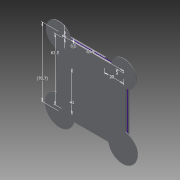
# Autodesk Inventor part: OuterCover
Saved by Autodesk Inventor 2014 SP1 (Build 180222100, 222)
## iProperties
Created: 2014-08-07
Part Number: OuterCover
Material: Generic
Document SubType Name: Modeling
Designer: Erin
Density: 1 g/cm^3
Appearance: Default
Author: Erin
Autodesk Inventor part; units mm, degrees
ref_plane "YZ Plane" through (0, 0, 0) normal (1, 0, 0) x (0, 1, 0)
ref_plane "XZ Plane" through (0, 0, 0) normal (0, 1, 0) x (-1, 0, 0)
ref_plane "XY Plane" through (0, 0, 0) normal (0, 0, 1) x (1, 0, 0)
sketch "Sketch1" plane through (0, 0, 0) normal (0, 1, 0) x (-1, 0, 0)
  line L0 (-31.75, 31.75) -> (31.75, 31.75)
  line L1 (31.75, 31.75) -> (31.75, -31.75)
  line L2 (31.75, -31.75) -> (-31.75, -31.75)
  line L3 (-31.75, -31.75) -> (-31.75, 31.75)
  line L4 (-31.75, 9.25) -> (31.75, 9.25) construction
  line L5 (-31.75, 26.75) -> (-11.75, 26.75) construction
  line L6 (-11.75, 26.75) -> (-11.75, 31.75) construction
  line L7 (32.35, 32.35) -> (-32.35, 32.35)
  line L8 (-32.35, 32.35) -> (-32.35, -32.35)
  line L9 (-32.35, -32.35) -> (32.35, -32.35)
  line L10 (32.35, -32.35) -> (32.35, 32.35)
  line L11 (-35.35, 35.35) -> (35.35, 35.35)
  line L12 (35.35, 35.35) -> (35.35, -35.35)
  line L13 (35.35, -35.35) -> (-35.35, -35.35)
  line L14 (-35.35, -35.35) -> (-35.35, 35.35)
  line L15 (-11.75, 31.75) -> (-31.75, 31.75)
  line L16 (-31.75, 31.75) -> (-31.75, 35.35)
  line L17 (-31.75, 35.35) -> (-11.75, 35.35)
  line L18 (-11.75, 35.35) -> (-11.75, 31.75)
  point P0 (0, 0)
  point P1 (0, 31.75)
  point P2 (31.75, 0)
  dimension "d0" = 63.5
  dimension "d1" = 63.5
  dimension "d2" = 41
  dimension "d3" = 5
  dimension "d4" = 20
  dimension "d6" = 3
  dimension "d7" = 0.6
  dimension "d17" = 70.7
  constraints: 38 end point, 9 parallel, 6 perpendicular, 5 point on line, 2 horizontal, 2 midpoint, 1 horizontal alignment, 1 vertical alignment, 6 other
  measures "d0" distance of L0.start L0.end
  measures "d1" distance of L0.end L1.end
  measures "d2" distance between parallel lines of L2 L4
  measures "d3" distance between parallel lines of L5 L0
  measures "d4" distance of L5.start L5.end
  measures "d6" distance between parallel lines of L7 L11
  measures "d7" distance between parallel lines of L0 L7
  measures "d17" distance between parallel lines of L13 L11
extrude "Extrusion1" add sketch "Sketch1" along normal blind 1.85 contours L7 L8 L9 L10 L18 L11 L12 L13 L14 L16
extrude "Extrusion3" add sketch "Sketch1" against normal blind 2
sketch "Sketch3" plane through (0, 0, 0) normal (0, 1, 0) x (1, 0, 0)
  line L0 (28.2668, -23.398) -> (-28.1063, -23.398) construction
  line L1 (-28.1063, -23.398) -> (-28.1063, -17.0805) construction
  line L2 (-28.1063, -17.0805) -> (28.2668, -17.0805) construction
  line L3 (28.2668, -17.0805) -> (28.2668, -23.398) construction
  line L4 (27.6672, -5.1215) -> (-28.7059, -5.1215) construction
  line L5 (-28.7059, -5.1215) -> (-28.7059, 1.196) construction
  line L6 (-28.7059, 1.196) -> (27.6672, 1.196) construction
  line L7 (27.6672, 1.196) -> (27.6672, -5.1215) construction
  spline S0 degree 2 poles (22.76, -19.0578) (22.76, -18.603) (23.1061, -17.9159) (23.3928, -17.6885) knots 0 0 0 1 2 2 2
  spline S1 degree 2 poles (23.3928, -17.6885) (23.7388, -17.4167) (24.5594, -17.1893) (25.1971, -17.1893) knots 0 0 0 1 2 2 2
  line L8 (25.1971, -17.1893) -> (27.6341, -17.1893)
  line L9 (27.6341, -17.1893) -> (27.6341, -23.2893)
  line L10 (27.6341, -23.2893) -> (25.4838, -23.2893)
  spline S2 degree 2 poles (25.4838, -23.2893) (24.8115, -23.2893) (24.1194, -23.1855) (23.8179, -23.0223) knots 0 0 0 1 2 2 2
  spline S3 degree 2 poles (23.8179, -23.0223) (23.4867, -22.8493) (23.1654, -22.2561) (23.1654, -21.8705) knots 0 0 0 1 2 2 2
  spline S4 degree 2 poles (23.1654, -21.8705) (23.1654, -21.4256) (23.6103, -20.7286) (24.0057, -20.5655) knots 0 0 0 1 2 2 2
  line L11 (24.0057, -20.5655) -> (24.0057, -20.5359)
  spline S5 degree 2 poles (24.0057, -20.5359) (23.4373, -20.4172) (22.76, -19.6807) (22.76, -19.0578) knots 0 0 0 1 2 2 2
  spline S6 degree 2 poles (24.3419, -19.0825) (24.3419, -19.3692) (24.5693, -19.6906) (24.7967, -19.7746) knots 0 0 0 1 2 2 2
  spline S7 degree 2 poles (24.7967, -19.7746) (24.9351, -19.829) (25.4245, -19.8389) (25.8298, -19.8389) knots 0 0 0 1 2 2 2
  line L12 (25.8298, -19.8389) -> (26.1116, -19.8389)
  line L13 (26.1116, -19.8389) -> (26.1116, -18.3015)
  line L14 (26.1116, -18.3015) -> (26.0275, -18.3015)
  spline S8 degree 2 poles (26.0275, -18.3015) (25.4343, -18.3015) (24.9796, -18.3163) (24.7423, -18.4201) knots 0 0 0 1 2 2 2
  spline S9 degree 2 poles (24.7423, -18.4201) (24.5347, -18.5141) (24.3419, -18.8601) (24.3419, -19.0825) knots 0 0 0 1 2 2 2
  spline S10 degree 2 poles (24.7225, -21.569) (24.7225, -21.7173) (24.8758, -22.0287) (25.0339, -22.0979) knots 0 0 0 1 2 2 2
  spline S11 degree 2 poles (25.0339, -22.0979) (25.1822, -22.1671) (25.5975, -22.177) (26.0078, -22.177) knots 0 0 0 1 2 2 2
  line L15 (26.0078, -22.177) -> (26.1116, -22.177)
  line L16 (26.1116, -22.177) -> (26.1116, -20.8819)
  line L17 (26.1116, -20.8819) -> (25.9188, -20.8819)
  spline S12 degree 2 poles (25.9188, -20.8819) (25.5283, -20.8819) (25.2119, -20.8967) (25.0438, -20.9758) knots 0 0 0 1 2 2 2
  spline S13 degree 2 poles (25.0438, -20.9758) (24.8609, -21.0648) (24.7225, -21.3663) (24.7225, -21.569) knots 0 0 0 1 2 2 2
  line L18 (21.8801, -17.1893) -> (21.8801, -23.2893)
  line L19 (21.8801, -23.2893) -> (17.7574, -23.2893)
  line L20 (17.7574, -23.2893) -> (17.7574, -22.1276)
  line L21 (17.7574, -22.1276) -> (20.3576, -22.1276)
  line L22 (20.3576, -22.1276) -> (20.3576, -21.0549)
  line L23 (20.3576, -21.0549) -> (17.9601, -21.0549)
  line L24 (17.9601, -21.0549) -> (17.9601, -19.8932)
  line L25 (17.9601, -19.8932) -> (20.3576, -19.8932)
  line L26 (20.3576, -19.8932) -> (20.3576, -18.3509)
  line L27 (20.3576, -18.3509) -> (17.7574, -18.3509)
  line L28 (17.7574, -18.3509) -> (17.7574, -17.1893)
  line L29 (17.7574, -17.1893) -> (21.8801, -17.1893)
  line L30 (11.2274, -17.1893) -> (14.5097, -17.1893)
  line L31 (14.5097, -17.1893) -> (14.5097, -18.2521)
  line L32 (14.5097, -18.2521) -> (13.6347, -18.2521)
  line L33 (13.6347, -18.2521) -> (13.6347, -22.2265)
  line L34 (13.6347, -22.2265) -> (14.5097, -22.2265)
  line L35 (14.5097, -22.2265) -> (14.5097, -23.2893)
  line L36 (14.5097, -23.2893) -> (11.2274, -23.2893)
  line L37 (11.2274, -23.2893) -> (11.2274, -22.2265)
  line L38 (11.2274, -22.2265) -> (12.1023, -22.2265)
  line L39 (12.1023, -22.2265) -> (12.1023, -18.2521)
  line L40 (12.1023, -18.2521) -> (11.2274, -18.2521)
  line L41 (11.2274, -18.2521) -> (11.2274, -17.1893)
  line L42 (4.984, -17.1893) -> (6.4571, -17.1893)
  line L43 (6.4571, -17.1893) -> (8.8101, -21.4405)
  line L44 (8.8101, -21.4405) -> (8.8101, -17.1893)
  line L45 (8.8101, -17.1893) -> (10.2091, -17.1893)
  line L46 (10.2091, -17.1893) -> (10.2091, -23.2893)
  line L47 (10.2091, -23.2893) -> (8.3306, -23.2893)
  line L48 (8.3306, -23.2893) -> (6.383, -19.7944)
  line L49 (6.383, -19.7944) -> (6.383, -23.2893)
  line L50 (6.383, -23.2893) -> (4.984, -23.2893)
  line L51 (4.984, -23.2893) -> (4.984, -17.1893)
  spline S14 degree 2 poles (1.8599, -17.0805) (2.5618, -17.0805) (3.6197, -17.3524) (4.0745, -17.5501) knots 0 0 0 1 2 2 2
  line L52 (4.0745, -17.5501) -> (4.0745, -19.0034)
  line L53 (4.0745, -19.0034) -> (3.936, -19.0034)
  spline S15 degree 2 poles (3.936, -19.0034) (3.4763, -18.6129) (2.374, -18.1927) (1.8549, -18.1927) knots 0 0 0 1 2 2 2
  spline S16 degree 2 poles (1.8549, -18.1927) (1.7215, -18.1927) (1.2914, -18.2521) (1.1629, -18.3114) knots 0 0 0 1 2 2 2
  spline S17 degree 2 poles (1.1629, -18.3114) (1.0047, -18.3806) (0.7822, -18.6327) (0.7822, -18.8354) knots 0 0 0 1 2 2 2
  spline S18 degree 2 poles (0.7822, -18.8354) (0.7822, -19.0677) (1.1431, -19.3544) (1.3903, -19.4187) knots 0 0 0 1 2 2 2
  spline S19 degree 2 poles (1.3903, -19.4187) (1.7017, -19.5027) (2.4086, -19.6461) (2.72, -19.7548) knots 0 0 0 1 2 2 2
  spline S20 degree 2 poles (2.72, -19.7548) (3.4269, -20.002) (4.0399, -20.8473) (4.0399, -21.48) knots 0 0 0 1 2 2 2
  spline S21 degree 2 poles (4.0399, -21.48) (4.0399, -22.3352) (2.5915, -23.398) (1.504, -23.398) knots 0 0 0 1 2 2 2
  spline S22 degree 2 poles (1.504, -23.398) (0.9602, -23.398) (-0.1174, -23.1756) (-0.5426, -22.9877) knots 0 0 0 1 2 2 2
  line L54 (-0.5426, -22.9877) -> (-0.5426, -21.5937)
  line L55 (-0.5426, -21.5937) -> (-0.4091, -21.5937)
  spline S23 degree 2 poles (-0.4091, -21.5937) (-0.068, -21.8854) (0.9108, -22.2858) (1.4249, -22.2858) knots 0 0 0 1 2 2 2
  spline S24 degree 2 poles (1.4249, -22.2858) (1.6275, -22.2858) (1.9439, -22.2265) (2.1219, -22.1474) knots 0 0 0 1 2 2 2
  spline S25 degree 2 poles (2.1219, -22.1474) (2.2652, -22.0831) (2.4728, -21.8261) (2.4728, -21.6679) knots 0 0 0 1 2 2 2
  spline S26 degree 2 poles (2.4728, -21.6679) (2.4728, -21.4306) (2.1416, -21.1587) (1.6671, -21.05) knots 0 0 0 1 2 2 2
  spline S27 degree 2 poles (1.6671, -21.05) (1.3606, -20.9808) (0.7921, -20.8473) (0.4659, -20.7336) knots 0 0 0 1 2 2 2
  spline S28 degree 2 poles (0.4659, -20.7336) (-0.1669, -20.5013) (-0.7848, -19.7301) (-0.7848, -19.0974) knots 0 0 0 1 2 2 2
  spline S29 degree 2 poles (-0.7848, -19.0974) (-0.7848, -18.1878) (0.6438, -17.0805) (1.8599, -17.0805) knots 0 0 0 1 2 2 2
  spline S30 degree 2 poles (-6.2619, -21.3663) (-6.2619, -20.9412) (-5.99, -20.1701) (-5.7379, -19.913) knots 0 0 0 1 2 2 2
  spline S31 degree 2 poles (-5.7379, -19.913) (-5.5847, -19.7499) (-5.209, -19.4829) (-4.9866, -19.389) knots 0 0 0 1 2 2 2
  spline S32 degree 2 poles (-4.9866, -19.389) (-4.7592, -19.2951) (-4.2302, -19.1863) (-3.904, -19.1863) knots 0 0 0 1 2 2 2
  line L56 (-3.904, -19.1863) -> (-3.1032, -19.1863)
  line L57 (-3.1032, -19.1863) -> (-3.1032, -17.1893)
  line L58 (-3.1032, -17.1893) -> (-1.5708, -17.1893)
  line L59 (-1.5708, -17.1893) -> (-1.5708, -23.2893)
  line L60 (-1.5708, -23.2893) -> (-3.9386, -23.2893)
  spline S33 degree 2 poles (-3.9386, -23.2893) (-4.4626, -23.2893) (-5.2288, -23.0965) (-5.5402, -22.8889) knots 0 0 0 1 2 2 2
  spline S34 degree 2 poles (-5.5402, -22.8889) (-5.8862, -22.6565) (-6.2619, -21.8953) (-6.2619, -21.3663) knots 0 0 0 1 2 2 2
  spline S35 degree 2 poles (-4.69, -21.3268) (-4.69, -21.5888) (-4.4428, -21.9595) (-4.2747, -22.0287) knots 0 0 0 1 2 2 2
  spline S36 degree 2 poles (-4.2747, -22.0287) (-4.0572, -22.1226) (-3.6618, -22.1523) (-3.3207, -22.1523) knots 0 0 0 1 2 2 2
  line L61 (-3.3207, -22.1523) -> (-3.1032, -22.1523)
  line L62 (-3.1032, -22.1523) -> (-3.1032, -20.3233)
  line L63 (-3.1032, -20.3233) -> (-3.2119, -20.3233)
  spline S37 degree 2 poles (-3.2119, -20.3233) (-3.4245, -20.3233) (-3.8101, -20.3332) (-3.9534, -20.3579) knots 0 0 0 1 2 2 2
  spline S38 degree 2 poles (-3.9534, -20.3579) (-4.077, -20.3777) (-4.3489, -20.4963) (-4.423, -20.5705) knots 0 0 0 1 2 2 2
  spline S39 degree 2 poles (-4.423, -20.5705) (-4.5812, -20.7188) (-4.69, -21.05) (-4.69, -21.3268) knots 0 0 0 1 2 2 2
  line L64 (-10.1177, -17.1893) -> (-6.8353, -17.1893)
  line L65 (-6.8353, -17.1893) -> (-6.8353, -18.2521)
  line L66 (-6.8353, -18.2521) -> (-7.7103, -18.2521)
  line L67 (-7.7103, -18.2521) -> (-7.7103, -22.2265)
  line L68 (-7.7103, -22.2265) -> (-6.8353, -22.2265)
  line L69 (-6.8353, -22.2265) -> (-6.8353, -23.2893)
  line L70 (-6.8353, -23.2893) -> (-10.1177, -23.2893)
  line L71 (-10.1177, -23.2893) -> (-10.1177, -22.2265)
  line L72 (-10.1177, -22.2265) -> (-9.2427, -22.2265)
  line L73 (-9.2427, -22.2265) -> (-9.2427, -18.2521)
  line L74 (-9.2427, -18.2521) -> (-10.1177, -18.2521)
  line L75 (-10.1177, -18.2521) -> (-10.1177, -17.1893)
  line L76 (-16.7713, -17.1893) -> (-14.9077, -17.1893)
  line L77 (-14.9077, -17.1893) -> (-13.2122, -19.4286)
  line L78 (-13.2122, -19.4286) -> (-12.6585, -19.4286)
  line L79 (-12.6585, -19.4286) -> (-12.6585, -17.1893)
  line L80 (-12.6585, -17.1893) -> (-11.136, -17.1893)
  line L81 (-11.136, -17.1893) -> (-11.136, -23.2893)
  line L82 (-11.136, -23.2893) -> (-13.5879, -23.2893)
  spline S40 degree 2 poles (-13.5879, -23.2893) (-14.097, -23.2893) (-14.8484, -23.1607) (-15.1697, -22.963) knots 0 0 0 1 2 2 2
  spline S41 degree 2 poles (-15.1697, -22.963) (-15.496, -22.7554) (-15.8815, -22.1078) (-15.8815, -21.6135) knots 0 0 0 1 2 2 2
  spline S42 degree 2 poles (-15.8815, -21.6135) (-15.8815, -20.9165) (-15.2488, -20.0415) (-14.7199, -19.7845) knots 0 0 0 1 2 2 2
  line L83 (-14.7199, -19.7845) -> (-16.7713, -17.1893)
  spline S43 degree 2 poles (-14.3096, -21.4207) (-14.3096, -21.653) (-14.1316, -21.9842) (-13.9289, -22.0732) knots 0 0 0 1 2 2 2
  spline S44 degree 2 poles (-13.9289, -22.0732) (-13.7856, -22.1325) (-13.4346, -22.1671) (-13.1726, -22.1671) knots 0 0 0 1 2 2 2
  line L84 (-13.1726, -22.1671) -> (-12.6585, -22.1671)
  line L85 (-12.6585, -22.1671) -> (-12.6585, -20.526)
  line L86 (-12.6585, -20.526) -> (-13.0985, -20.526)
  spline S45 degree 2 poles (-13.0985, -20.526) (-13.4148, -20.526) (-13.8647, -20.6051) (-14.0179, -20.7286) knots 0 0 0 1 2 2 2
  spline S46 degree 2 poles (-14.0179, -20.7286) (-14.1662, -20.8473) (-14.3096, -21.1637) (-14.3096, -21.4207) knots 0 0 0 1 2 2 2
  line L87 (-17.2261, -17.1893) -> (-17.2261, -23.2893)
  line L88 (-17.2261, -23.2893) -> (-21.3488, -23.2893)
  line L89 (-21.3488, -23.2893) -> (-21.3488, -22.1276)
  line L90 (-21.3488, -22.1276) -> (-18.7486, -22.1276)
  line L91 (-18.7486, -22.1276) -> (-18.7486, -21.0549)
  line L92 (-18.7486, -21.0549) -> (-21.1461, -21.0549)
  line L93 (-21.1461, -21.0549) -> (-21.1461, -19.8932)
  line L94 (-21.1461, -19.8932) -> (-18.7486, -19.8932)
  line L95 (-18.7486, -19.8932) -> (-18.7486, -18.3509)
  line L96 (-18.7486, -18.3509) -> (-21.3488, -18.3509)
  line L97 (-21.3488, -18.3509) -> (-21.3488, -17.1893)
  line L98 (-21.3488, -17.1893) -> (-17.2261, -17.1893)
  spline S47 degree 2 poles (-27.8294, -20.2343) (-27.8294, -19.3791) (-27.083, -18.0346) (-26.5145, -17.6737) knots 0 0 0 1 2 2 2
  spline S48 degree 2 poles (-26.5145, -17.6737) (-26.04, -17.3672) (-24.9228, -17.1893) (-24.295, -17.1893) knots 0 0 0 1 2 2 2
  line L99 (-24.295, -17.1893) -> (-22.3869, -17.1893)
  line L100 (-22.3869, -17.1893) -> (-22.3869, -23.2893)
  line L101 (-22.3869, -23.2893) -> (-24.2752, -23.2893)
  spline S49 degree 2 poles (-24.2752, -23.2893) (-24.9178, -23.2893) (-26.04, -23.1261) (-26.5343, -22.8098) knots 0 0 0 1 2 2 2
  spline S50 degree 2 poles (-26.5343, -22.8098) (-27.1324, -22.4242) (-27.8294, -21.1192) (-27.8294, -20.2343) knots 0 0 0 1 2 2 2
  spline S51 degree 2 poles (-26.2575, -20.2442) (-26.2575, -20.8473) (-25.8422, -21.7074) (-25.4171, -21.9496) knots 0 0 0 1 2 2 2
  spline S52 degree 2 poles (-25.4171, -21.9496) (-25.1057, -22.1177) (-24.4235, -22.1523) (-23.949, -22.1523) knots 0 0 0 1 2 2 2
  line L102 (-23.949, -22.1523) -> (-23.9193, -22.1523)
  line L103 (-23.9193, -22.1523) -> (-23.9193, -18.3312)
  line L104 (-23.9193, -18.3312) -> (-23.949, -18.3312)
  spline S53 degree 2 poles (-23.949, -18.3312) (-24.4631, -18.3312) (-25.17, -18.3658) (-25.4913, -18.5684) knots 0 0 0 1 2 2 2
  spline S54 degree 2 poles (-25.4913, -18.5684) (-25.867, -18.8057) (-26.2575, -19.6411) (-26.2575, -20.2442) knots 0 0 0 1 2 2 2
  spline S55 degree 2 poles (12.6643, 1.2157) (14.0386, 1.2157) (15.6501, -0.4452) (15.6501, -1.948) knots 0 0 0 1 2 2 2
  spline S56 degree 2 poles (15.6501, -1.948) (15.6501, -3.3963) (14.0336, -5.1215) (12.6594, -5.1215) knots 0 0 0 1 2 2 2
  spline S57 degree 2 poles (12.6594, -5.1215) (12.2985, -5.1215) (11.7152, -5.0375) (11.4483, -4.9683) knots 0 0 0 1 2 2 2
  spline S58 degree 2 poles (11.4483, -4.9683) (11.2407, -4.904) (10.7513, -4.6915) (10.598, -4.6124) knots 0 0 0 1 2 2 2
  line L105 (10.598, -4.6124) -> (10.598, -3.1591)
  line L106 (10.598, -3.1591) -> (10.7513, -3.1591)
  spline S59 degree 2 poles (10.7513, -3.1591) (10.865, -3.2579) (11.2011, -3.5348) (11.4137, -3.6633) knots 0 0 0 1 2 2 2
  spline S60 degree 2 poles (11.4137, -3.6633) (11.6262, -3.7967) (12.1354, -3.9796) (12.4172, -3.9796) knots 0 0 0 1 2 2 2
  spline S61 degree 2 poles (12.4172, -3.9796) (12.7484, -3.9796) (13.2971, -3.772) (13.5492, -3.51) knots 0 0 0 1 2 2 2
  spline S62 degree 2 poles (13.5492, -3.51) (13.7766, -3.2777) (14.0682, -2.4818) (14.0682, -1.943) knots 0 0 0 1 2 2 2
  spline S63 degree 2 poles (14.0682, -1.943) (14.0682, -1.3745) (13.7667, -0.5984) (13.5195, -0.3612) knots 0 0 0 1 2 2 2
  spline S64 degree 2 poles (13.5195, -0.3612) (13.2822, -0.1288) (12.6989, 0.0738) (12.4073, 0.0738) knots 0 0 0 1 2 2 2
  spline S65 degree 2 poles (12.4073, 0.0738) (12.1057, 0.0738) (11.557, -0.1288) (11.3692, -0.2524) knots 0 0 0 1 2 2 2
  spline S66 degree 2 poles (11.3692, -0.2524) (11.1616, -0.376) (10.8501, -0.638) (10.7365, -0.7418) knots 0 0 0 1 2 2 2
  line L107 (10.7365, -0.7418) -> (10.598, -0.7418)
  line L108 (10.598, -0.7418) -> (10.598, 0.6917)
  spline S67 degree 2 poles (10.598, 0.6917) (10.7661, 0.7708) (11.2061, 0.9686) (11.4433, 1.0378) knots 0 0 0 1 2 2 2
  spline S68 degree 2 poles (11.4433, 1.0378) (11.7301, 1.1268) (12.2293, 1.2157) (12.6643, 1.2157) knots 0 0 0 1 2 2 2
  line L109 (4.0581, 1.0971) -> (5.9217, 1.0971)
  line L110 (5.9217, 1.0971) -> (7.6172, -1.1422)
  line L111 (7.6172, -1.1422) -> (8.1709, -1.1422)
  line L112 (8.1709, -1.1422) -> (8.1709, 1.0971)
  line L113 (8.1709, 1.0971) -> (9.6934, 1.0971)
  line L114 (9.6934, 1.0971) -> (9.6934, -5.0029)
  line L115 (9.6934, -5.0029) -> (7.2416, -5.0029)
  spline S69 degree 2 poles (7.2416, -5.0029) (6.7324, -5.0029) (5.981, -4.8744) (5.6597, -4.6767) knots 0 0 0 1 2 2 2
  spline S70 degree 2 poles (5.6597, -4.6767) (5.3335, -4.469) (4.9479, -3.8215) (4.9479, -3.3271) knots 0 0 0 1 2 2 2
  spline S71 degree 2 poles (4.9479, -3.3271) (4.9479, -2.6301) (5.5806, -1.7552) (6.1095, -1.4981) knots 0 0 0 1 2 2 2
  line L116 (6.1095, -1.4981) -> (4.0581, 1.0971)
  spline S72 degree 2 poles (6.5198, -3.1343) (6.5198, -3.3667) (6.6978, -3.6979) (6.9005, -3.7869) knots 0 0 0 1 2 2 2
  spline S73 degree 2 poles (6.9005, -3.7869) (7.0438, -3.8462) (7.3948, -3.8808) (7.6568, -3.8808) knots 0 0 0 1 2 2 2
  line L117 (7.6568, -3.8808) -> (8.1709, -3.8808)
  line L118 (8.1709, -3.8808) -> (8.1709, -2.2396)
  line L119 (8.1709, -2.2396) -> (7.7309, -2.2396)
  spline S74 degree 2 poles (7.7309, -2.2396) (7.4146, -2.2396) (6.9647, -2.3187) (6.8115, -2.4423) knots 0 0 0 1 2 2 2
  spline S75 degree 2 poles (6.8115, -2.4423) (6.6632, -2.5609) (6.5198, -2.8773) (6.5198, -3.1343) knots 0 0 0 1 2 2 2
  line L120 (3.6033, 1.0971) -> (3.6033, -5.0029)
  line L121 (3.6033, -5.0029) -> (-0.5194, -5.0029)
  line L122 (-0.5194, -5.0029) -> (-0.5194, -3.8412)
  line L123 (-0.5194, -3.8412) -> (2.0808, -3.8412)
  line L124 (2.0808, -3.8412) -> (2.0808, -2.7685)
  line L125 (2.0808, -2.7685) -> (-0.3167, -2.7685)
  line L126 (-0.3167, -2.7685) -> (-0.3167, -1.6069)
  line L127 (-0.3167, -1.6069) -> (2.0808, -1.6069)
  line L128 (2.0808, -1.6069) -> (2.0808, -0.0646)
  line L129 (2.0808, -0.0646) -> (-0.5194, -0.0646)
  line L130 (-0.5194, -0.0646) -> (-0.5194, 1.0971)
  line L131 (-0.5194, 1.0971) -> (3.6033, 1.0971)
  line L132 (-0.9, 1.0971) -> (-2.9614, -5.0029)
  line L133 (-2.9614, -5.0029) -> (-4.6322, -5.0029)
  line L134 (-4.6322, -5.0029) -> (-6.6935, 1.0971)
  line L135 (-6.6935, 1.0971) -> (-5.1166, 1.0971)
  line L136 (-5.1166, 1.0971) -> (-4.736, -0.1486)
  line L137 (-4.736, -0.1486) -> (-2.818, -0.1486)
  line L138 (-2.818, -0.1486) -> (-2.4324, 1.0971)
  line L139 (-2.4324, 1.0971) -> (-0.9, 1.0971)
  line L140 (-4.3999, -1.2559) -> (-3.777, -3.2728)
  line L141 (-3.777, -3.2728) -> (-3.1492, -1.2559)
  line L142 (-3.1492, -1.2559) -> (-4.3999, -1.2559)
  line L143 (-8.4731, 1.0971) -> (-8.4731, -3.8412)
  line L144 (-8.4731, -3.8412) -> (-6.6688, -3.8412)
  line L145 (-6.6688, -3.8412) -> (-6.6688, -5.0029)
  line L146 (-6.6688, -5.0029) -> (-11.8098, -5.0029)
  line L147 (-11.8098, -5.0029) -> (-11.8098, -3.8412)
  line L148 (-11.8098, -3.8412) -> (-10.0055, -3.8412)
  line L149 (-10.0055, -3.8412) -> (-10.0055, 1.0971)
  line L150 (-10.0055, 1.0971) -> (-8.4731, 1.0971)
  line L151 (-12.4376, 1.0971) -> (-12.4376, -5.0029)
  line L152 (-12.4376, -5.0029) -> (-16.5603, -5.0029)
  line L153 (-16.5603, -5.0029) -> (-16.5603, -3.8412)
  line L154 (-16.5603, -3.8412) -> (-13.9601, -3.8412)
  line L155 (-13.9601, -3.8412) -> (-13.9601, -2.7685)
  line L156 (-13.9601, -2.7685) -> (-16.3576, -2.7685)
  line L157 (-16.3576, -2.7685) -> (-16.3576, -1.6069)
  line L158 (-16.3576, -1.6069) -> (-13.9601, -1.6069)
  line L159 (-13.9601, -1.6069) -> (-13.9601, -0.0646)
  line L160 (-13.9601, -0.0646) -> (-16.5603, -0.0646)
  line L161 (-16.5603, -0.0646) -> (-16.5603, 1.0971)
  line L162 (-16.5603, 1.0971) -> (-12.4376, 1.0971)
  line L163 (6.0305, 11.1406) -> (6.0305, 6.2023)
  line L164 (6.0305, 6.2023) -> (7.8348, 6.2023)
  line L165 (7.8348, 6.2023) -> (7.8348, 5.0406)
  line L166 (7.8348, 5.0406) -> (2.6937, 5.0406)
  line L167 (2.6937, 5.0406) -> (2.6937, 6.2023)
  line L168 (2.6937, 6.2023) -> (4.498, 6.2023)
  line L169 (4.498, 6.2023) -> (4.498, 11.1406)
  line L170 (4.498, 11.1406) -> (6.0305, 11.1406)
  line L171 (-3.08, 11.1406) -> (-1.5476, 11.1406)
  line L172 (-1.5476, 11.1406) -> (-1.5476, 8.4366)
  line L173 (-1.5476, 8.4366) -> (0.5335, 8.4366)
  line L174 (0.5335, 8.4366) -> (0.5335, 11.1406)
  line L175 (0.5335, 11.1406) -> (2.066, 11.1406)
  line L176 (2.066, 11.1406) -> (2.066, 5.0406)
  line L177 (2.066, 5.0406) -> (0.5335, 5.0406)
  line L178 (0.5335, 5.0406) -> (0.5335, 7.2749)
  line L179 (0.5335, 7.2749) -> (-1.5476, 7.2749)
  line L180 (-1.5476, 7.2749) -> (-1.5476, 5.0406)
  line L181 (-1.5476, 5.0406) -> (-3.08, 5.0406)
  line L182 (-3.08, 5.0406) -> (-3.08, 11.1406)
  line L183 (-4.3455, 11.1406) -> (-4.3455, 5.0406)
  line L184 (-4.3455, 5.0406) -> (-8.4682, 5.0406)
  line L185 (-8.4682, 5.0406) -> (-8.4682, 6.2023)
  line L186 (-8.4682, 6.2023) -> (-5.868, 6.2023)
  line L187 (-5.868, 6.2023) -> (-5.868, 7.2749)
  line L188 (-5.868, 7.2749) -> (-8.2655, 7.2749)
  line L189 (-8.2655, 7.2749) -> (-8.2655, 8.4366)
  line L190 (-8.2655, 8.4366) -> (-5.868, 8.4366)
  line L191 (-5.868, 8.4366) -> (-5.868, 9.9789)
  line L192 (-5.868, 9.9789) -> (-8.4682, 9.9789)
  line L193 (-8.4682, 9.9789) -> (-8.4682, 11.1406)
  line L194 (-8.4682, 11.1406) -> (-4.3455, 11.1406)
  line L195 (11.5941, 16.2457) -> (14.1547, 16.2457)
  line L196 (14.1547, 16.2457) -> (14.1547, 17.3975)
  line L197 (14.1547, 17.3975) -> (11.7968, 17.3975)
  line L198 (11.7968, 17.3975) -> (11.7968, 18.5592)
  line L199 (11.7968, 18.5592) -> (14.1547, 18.5592)
  line L200 (14.1547, 18.5592) -> (14.1547, 21.1841)
  line L201 (14.1547, 21.1841) -> (15.6773, 21.1841)
  line L202 (15.6773, 21.1841) -> (15.6773, 15.0841)
  line L203 (15.6773, 15.0841) -> (11.5941, 15.0841)
  line L204 (11.5941, 15.0841) -> (11.5941, 16.2457)
  spline S76 degree 2 poles (8.3365, 21.3126) (9.5674, 21.3126) (10.8922, 20.1262) (10.8922, 18.9794) knots 0 0 0 1 2 2 2
  line L205 (10.8922, 18.9794) -> (10.8922, 15.0841)
  line L206 (10.8922, 15.0841) -> (9.3598, 15.0841)
  line L207 (9.3598, 15.0841) -> (9.3598, 18.8904)
  spline S77 degree 2 poles (9.3598, 18.8904) (9.3598, 19.5281) (8.8803, 20.1509) (8.3365, 20.1509) knots 0 0 0 1 2 2 2
  spline S78 degree 2 poles (8.3365, 20.1509) (7.8076, 20.1509) (7.3132, 19.5528) (7.3132, 18.8904) knots 0 0 0 1 2 2 2
  line L208 (7.3132, 18.8904) -> (7.3132, 15.0841)
  line L209 (7.3132, 15.0841) -> (5.7808, 15.0841)
  line L210 (5.7808, 15.0841) -> (5.7808, 18.9744)
  spline S79 degree 2 poles (5.7808, 18.9744) (5.7808, 20.1015) (7.071, 21.3126) (8.3365, 21.3126) knots 0 0 0 1 2 2 2
  line L211 (3.4328, 21.1841) -> (3.4328, 16.2457)
  line L212 (3.4328, 16.2457) -> (5.2371, 16.2457)
  line L213 (5.2371, 16.2457) -> (5.2371, 15.0841)
  line L214 (5.2371, 15.0841) -> (0.0961, 15.0841)
  line L215 (0.0961, 15.0841) -> (0.0961, 16.2457)
  line L216 (0.0961, 16.2457) -> (1.9004, 16.2457)
  line L217 (1.9004, 16.2457) -> (1.9004, 21.1841)
  line L218 (1.9004, 21.1841) -> (3.4328, 21.1841)
  spline S80 degree 2 poles (-2.9984, 21.3126) (-1.7676, 21.3126) (-0.4428, 20.1262) (-0.4428, 18.9794) knots 0 0 0 1 2 2 2
  line L219 (-0.4428, 18.9794) -> (-0.4428, 15.0841)
  line L220 (-0.4428, 15.0841) -> (-1.9752, 15.0841)
  line L221 (-1.9752, 15.0841) -> (-1.9752, 18.8904)
  spline S81 degree 2 poles (-1.9752, 18.8904) (-1.9752, 19.5281) (-2.4547, 20.1509) (-2.9984, 20.1509) knots 0 0 0 1 2 2 2
  spline S82 degree 2 poles (-2.9984, 20.1509) (-3.5274, 20.1509) (-4.0217, 19.5528) (-4.0217, 18.8904) knots 0 0 0 1 2 2 2
  line L222 (-4.0217, 18.8904) -> (-4.0217, 15.0841)
  line L223 (-4.0217, 15.0841) -> (-5.5541, 15.0841)
  line L224 (-5.5541, 15.0841) -> (-5.5541, 18.9744)
  spline S83 degree 2 poles (-5.5541, 18.9744) (-5.5541, 20.1015) (-4.2639, 21.3126) (-2.9984, 21.3126) knots 0 0 0 1 2 2 2
  line L225 (-12.3659, 21.1841) -> (-10.5023, 21.1841)
  line L226 (-10.5023, 21.1841) -> (-8.8068, 18.9448)
  line L227 (-8.8068, 18.9448) -> (-8.2531, 18.9448)
  line L228 (-8.2531, 18.9448) -> (-8.2531, 21.1841)
  line L229 (-8.2531, 21.1841) -> (-6.7306, 21.1841)
  line L230 (-6.7306, 21.1841) -> (-6.7306, 15.0841)
  line L231 (-6.7306, 15.0841) -> (-9.1825, 15.0841)
  spline S84 degree 2 poles (-9.1825, 15.0841) (-9.6916, 15.0841) (-10.443, 15.2126) (-10.7643, 15.4103) knots 0 0 0 1 2 2 2
  spline S85 degree 2 poles (-10.7643, 15.4103) (-11.0906, 15.6179) (-11.4761, 16.2655) (-11.4761, 16.7598) knots 0 0 0 1 2 2 2
  spline S86 degree 2 poles (-11.4761, 16.7598) (-11.4761, 17.4568) (-10.8434, 18.3318) (-10.3145, 18.5889) knots 0 0 0 1 2 2 2
  line L232 (-10.3145, 18.5889) -> (-12.3659, 21.1841)
  spline S87 degree 2 poles (-9.9042, 16.9526) (-9.9042, 16.7203) (-9.7262, 16.3891) (-9.5236, 16.3001) knots 0 0 0 1 2 2 2
  spline S88 degree 2 poles (-9.5236, 16.3001) (-9.3802, 16.2408) (-9.0292, 16.2062) (-8.7672, 16.2062) knots 0 0 0 1 2 2 2
  line L233 (-8.7672, 16.2062) -> (-8.2531, 16.2062)
  line L234 (-8.2531, 16.2062) -> (-8.2531, 17.8474)
  line L235 (-8.2531, 17.8474) -> (-8.6931, 17.8474)
  spline S89 degree 2 poles (-8.6931, 17.8474) (-9.0095, 17.8474) (-9.4593, 17.7683) (-9.6125, 17.6447) knots 0 0 0 1 2 2 2
  spline S90 degree 2 poles (-9.6125, 17.6447) (-9.7608, 17.5261) (-9.9042, 17.2097) (-9.9042, 16.9526) knots 0 0 0 1 2 2 2
  line L236 (-12.8207, 21.1841) -> (-12.8207, 15.0841)
  line L237 (-12.8207, 15.0841) -> (-16.9434, 15.0841)
  line L238 (-16.9434, 15.0841) -> (-16.9434, 16.2457)
  line L239 (-16.9434, 16.2457) -> (-14.3432, 16.2457)
  line L240 (-14.3432, 16.2457) -> (-14.3432, 17.3184)
  line L241 (-14.3432, 17.3184) -> (-16.7407, 17.3184)
  line L242 (-16.7407, 17.3184) -> (-16.7407, 18.4801)
  line L243 (-16.7407, 18.4801) -> (-14.3432, 18.4801)
  line L244 (-14.3432, 18.4801) -> (-14.3432, 20.0224)
  line L245 (-14.3432, 20.0224) -> (-16.9434, 20.0224)
  line L246 (-16.9434, 20.0224) -> (-16.9434, 21.1841)
  line L247 (-16.9434, 21.1841) -> (-12.8207, 21.1841)
  point P0 (0, 0)
  constraints: 4 other
extrude "Extrusion4" cut sketch "Sketch3" against normal blind 1
sketch "Sketch4" plane through (0, -2, 0) normal (0, -1, 0) x (1, 0, 0)
  circle A0 centre (-33.444, 33.5438) radius 12.9475
  circle A1 centre (-32.4457, -32.5455) radius 15.0082
  point P0 (0, 0)
  constraints: 2 centre point
extrude "Extrusion5" add sketch "Sketch4" against normal blind 0.6
mirror "Mirror1" about plane through (0, 0, 0) normal (1, 0, 0) of "Extrusion5"
body "Solid1"
